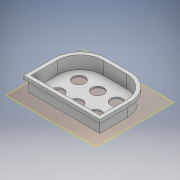
# Autodesk Inventor part: bottleHolder
Saved by Autodesk Inventor 2017 (Build 210142000, 142)
## iProperties
Created: 2016-11-02
Part Number: bottleHolder
Material: Generic
Document SubType Name: Modeling
Designer: Camilo
Density: 1 g/cm^3
Appearance: Default
Author: Camilo
Autodesk Inventor part; units mm, degrees
ref_plane "YZ Plane" through (0, 0, 0) normal (1, 0, 0) x (0, 1, 0)
ref_plane "XZ Plane" through (0, 0, 0) normal (0, 1, 0) x (-1, 0, 0)
ref_plane "Work Plane1" through (0, 0, -20) normal (0, 0, 1) x (1, 0, 0)
sketch "Sketch1" plane through (0, 0, -20) normal (0, 0, 1) x (1, 0, 0)
  arc A0 (-24.5816, 56) -> (-77, 3.5816) centre (-24.5816, 3.5816) ccw construction
  line L0 (-24.5816, 56) -> (24.5816, 56) construction
  arc A1 (77, 3.5816) -> (24.5816, 56) centre (24.5816, 3.5816) ccw construction
  line L1 (77, 3.5816) -> (77, -56) construction
  line L2 (77, -56) -> (-77, -56) construction
  line L3 (-77, -56) -> (-77, 3.5816) construction
  line L4 (87, 75) -> (-87, 75) construction
  line L5 (-87, 75) -> (-87, -75) construction
  line L6 (-87, -75) -> (87, -75) construction
  line L7 (87, -75) -> (87, 75) construction
  line L8 (24.5816, 54.75) -> (-24.5816, 54.75)
  arc A2 (-24.5816, 54.75) -> (-75.75, 3.5816) centre (-24.5816, 3.5816) ccw
  line L9 (-75.75, 3.5816) -> (-75.75, -54.75)
  line L10 (-75.75, -54.75) -> (75.75, -54.75)
  line L11 (75.75, -54.75) -> (75.75, 3.5816)
  arc A3 (75.75, 3.5816) -> (24.5816, 54.75) centre (24.5816, 3.5816) ccw
  point P0 (0, 0)
  dimension "d0" = 1.25
  constraints: 8 end point, 4 point on circle, 2 centre point, 5 other
  measures "d0" distance between parallel lines of L2 L10
extrude "Extrusion1" add sketch "Sketch1" along normal blind 5
sketch "Sketch2" plane through (0, 0, -15) normal (0, 0, 1) x (1, 0, 0)
  line L0 (24.5816, 54.75) -> (-24.5816, 54.75) projected
  arc A0 (-24.5816, 54.75) -> (-75.75, 3.5816) centre (-24.5816, 3.5816) ccw projected
  line L1 (-75.75, 3.5816) -> (-75.75, -54.75) projected
  line L2 (-75.75, -54.75) -> (75.75, -54.75) projected
  line L3 (75.75, -54.75) -> (75.75, 3.5816) projected
  arc A1 (75.75, 3.5816) -> (24.5816, 54.75) centre (24.5816, 3.5816) ccw projected
  line L4 (24.5816, 52.25) -> (-24.5816, 52.25)
  arc A2 (-24.5816, 52.25) -> (-73.25, 3.5816) centre (-24.5816, 3.5816) ccw
  line L5 (-73.25, 3.5816) -> (-73.25, -52.25)
  line L6 (-73.25, -52.25) -> (73.25, -52.25)
  line L7 (73.25, -52.25) -> (73.25, 3.5816)
  arc A3 (73.25, 3.5816) -> (24.5816, 52.25) centre (24.5816, 3.5816) ccw
  point P0 (0, 0)
  dimension "d3" = 2.5
  constraints: 8 end point, 4 point on circle, 2 centre point, 5 other
  measures "d3" distance between parallel lines of L2 L6
ref_plane "Work Plane2" through (-87, -75, 0) normal (0, 0, 1) x (1, 0, 0)
extrude "Extrusion2" add sketch "Sketch2" along normal up to surface (15 mm away)
sketch "Sketch3" plane through (-75.75, -54.75, 0) normal (0, 0, 1) x (1, 0, 0)
  arc A0 (149, 58.3316) -> (100.3316, 107) centre (100.3316, 58.3316) ccw projected
  line L0 (149, 2.5) -> (149, 58.3316) projected
  line L1 (2.5, 2.5) -> (149, 2.5) projected
  line L2 (2.5, 58.3316) -> (2.5, 2.5) projected
  arc A1 (51.1684, 107) -> (2.5, 58.3316) centre (51.1684, 58.3316) ccw projected
  line L3 (100.3316, 107) -> (51.1684, 107) projected
  arc A2 (151.5, 58.3316) -> (100.3316, 109.5) centre (100.3316, 58.3316) ccw projected
  line L4 (51.1684, 109.5) -> (100.3316, 109.5) projected
  arc A3 (51.1684, 109.5) -> (0, 58.3316) centre (51.1684, 58.3316) ccw projected
  line L5 (0, 0) -> (0, 58.3316) projected
  line L6 (151.5, 0) -> (0, 0) projected
  line L7 (151.5, 58.3316) -> (151.5, 0) projected
  point P0 (75.75, 54.75)
extrude "Extrusion3" add sketch "Sketch3" along normal blind 5
sketch "Sketch4" plane through (-75.75, -54.75, 5) normal (0, 0, 1) x (1, 0, 0)
  line L0 (149, 58.3316) -> (149, 2.5) projected
  line L1 (149, 2.5) -> (2.5, 2.5) projected
  line L2 (2.5, 2.5) -> (2.5, 58.3316) projected
  arc A0 (51.1684, 107) -> (2.5, 58.3316) centre (51.1684, 58.3316) ccw projected
  line L3 (51.1684, 107) -> (100.3316, 107) projected
  arc A1 (149, 58.3316) -> (100.3316, 107) centre (100.3316, 58.3316) ccw projected
  arc A2 (151.5, 58.3316) -> (100.3316, 109.5) centre (100.3316, 58.3316) ccw construction
  line L4 (100.3316, 109.5) -> (51.1684, 109.5) construction
  arc A3 (51.1684, 109.5) -> (0, 58.3316) centre (51.1684, 58.3316) ccw construction
  line L5 (0, 58.3316) -> (0, 0) construction
  line L6 (0, 0) -> (151.5, 0) construction
  line L7 (151.5, 0) -> (151.5, 58.3316) construction
  line L8 (156.5, -5) -> (-5, -5)
  line L9 (-5, -5) -> (-5, 58.3316)
  arc A4 (51.1684, 114.5) -> (-5, 58.3316) centre (51.1684, 58.3316) ccw
  line L10 (51.1684, 114.5) -> (100.3316, 114.5)
  arc A5 (156.5, 58.3316) -> (100.3316, 114.5) centre (100.3316, 58.3316) ccw
  line L11 (156.5, 58.3316) -> (156.5, -5)
  point P0 (75.75, 54.75)
  dimension "d8" = 5
  constraints: 8 end point, 4 point on circle, 2 centre point, 5 other
  measures "d8" distance between parallel lines of L8 L6
extrude "Extrusion4" add sketch "Sketch4" along normal blind 2.5
chamfer "Chamfer1" distance 5 angle 45 6 edges at (-75.75, -25.5842, 5) (-60.7631, 39.7631, 5) (0, 54.75, 5) (60.7631, 39.7631, 5) (75.75, -25.5842, 5) (0, -54.75, 5)
sketch "Sketch5" plane through (0, 0, -15) normal (0, 0, 1) x (1, 0, 0)
  circle A0 centre (-41.25, -27.25) radius 12.75
  line L0 (-73.25, 3.5816) -> (-73.25, -52.25) projected
  line L1 (-73.25, -52.25) -> (73.25, -52.25) projected
  line L2 (73.25, -52.25) -> (73.25, 3.5816) projected
  arc A1 (73.25, 3.5816) -> (24.5816, 52.25) centre (24.5816, 3.5816) ccw projected
  line L3 (24.5816, 52.25) -> (-24.5816, 52.25) projected
  arc A2 (-24.5816, 52.25) -> (-73.25, 3.5816) centre (-24.5816, 3.5816) ccw projected
  circle A3 centre (-41.25, 17.75) radius 12.75
  circle A4 centre (-1.25, -27.25) radius 12.75
  circle A5 centre (-1.25, 17.75) radius 12.75
  circle A6 centre (38.75, -27.25) radius 12.75
  circle A7 centre (38.75, 17.75) radius 12.75
  point P0 (0, 0)
  dimension "d14" = 25.5
  dimension "d15" = 25
  dimension "d16" = 32
  dimension "d19" = 45
  dimension "d22" = 40
  constraints: 6 centre point, 1 horizontal, 1 vertical, 10 other
  measures "d14" diameter of A0
  measures "d15" distance from line of L1 A0.centre
  measures "d16" distance from line of A0.centre L0
  measures "d19" distance of A0.centre A3.centre
  measures "d22" distance of A0.centre A4.centre
extrude "Extrusion5" cut sketch "Sketch5" against normal through all contours A0 | A3 | A4 | A5 | A6 | A7
fillet "Fillet1" radius 2 6 edges at (26, -27.25, -20) (26, 17.75, -20) (-14, -27.25, -20) (-14, 17.75, -20) (-54, -27.25, -20) (-54, 17.75, -20)
fillet "Fillet2" radius 2 6 edges at (60.7631, 39.7631, -20) (0, 54.75, -20) (-60.7631, 39.7631, -20) (-75.75, -25.5842, -20) (75.75, -25.5842, -20) (0, -54.75, -20)
sketch "Sketch6" plane through (-75.75, -54.75, 7.5) normal (0, 0, 1) x (1, 0, 0)
  line L0 (149, 2.5) -> (2.5, 2.5) projected
  line L1 (2.5, 2.5) -> (2.5, 58.3316) projected
  arc A0 (51.1684, 107) -> (2.5, 58.3316) centre (51.1684, 58.3316) ccw projected
  line L2 (51.1684, 107) -> (100.3316, 107) projected
  arc A1 (149, 58.3316) -> (100.3316, 107) centre (100.3316, 58.3316) ccw projected
  line L3 (149, 58.3316) -> (149, 2.5) projected
  line L4 (-5, -5) -> (156.5, -5) projected
  line L5 (156.5, -5) -> (156.5, 58.3316) projected
  arc A2 (156.5, 58.3316) -> (100.3316, 114.5) centre (100.3316, 58.3316) ccw projected
  line L6 (100.3316, 114.5) -> (51.1684, 114.5) projected
  arc A3 (51.1684, 114.5) -> (-5, 58.3316) centre (51.1684, 58.3316) ccw projected
  line L7 (-5, 58.3316) -> (-5, -5) projected
  point P0 (75.75, 54.75)
extrude "Extrusion6" add sketch "Sketch6" along normal blind 5
body "Solid1"
